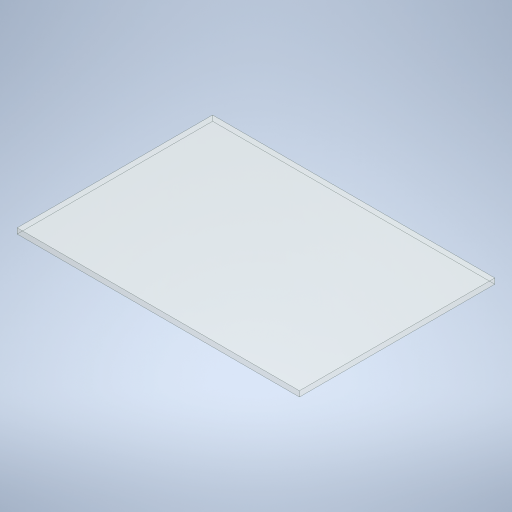
# Autodesk Inventor part: panel_13x9
Saved by Autodesk Inventor 2024 (Build 280153000, 153)
## iProperties
Created: 2024-09-19
Part Number: panel_13x9
Material: Glass
Document SubType Name: Modeling
Designer: Owner
Density: 2.18 g/cm^3
Appearance: Clear
Author: Owner
Autodesk Inventor part; units mm, degrees
ref_plane "YZ Plane" through (0, 0, 0) normal (1, 0, 0) x (0, 1, 0)
ref_plane "XZ Plane" through (0, 0, 0) normal (0, 1, 0) x (-1, 0, 0)
ref_plane "XY Plane" through (0, 0, 0) normal (0, 0, 1) x (1, 0, 0)
sketch "Sketch1" plane through (0, 0, 0) normal (0, 1, 0) x (-1, 0, 0)
  line L0 (165.1, 114.3) -> (-165.1, 114.3)
  line L1 (-165.1, 114.3) -> (-165.1, -114.3)
  line L2 (-165.1, -114.3) -> (165.1, -114.3)
  line L3 (165.1, -114.3) -> (165.1, 114.3)
  line L4 (165.1, 114.3) -> (-165.1, -114.3) construction
  line L5 (-165.1, 114.3) -> (165.1, -114.3) construction
  point P0 (0, 0)
  dimension "d0" = 330.2
  dimension "d1" = 228.6
  constraints: 12 end point, 2 midpoint, 2 parallel, 1 horizontal, 1 perpendicular
  measures "d0" distance of L2.end L1.end
  measures "d1" distance of L1.end L0.end
extrude "Extrusion1" add sketch "Sketch1" along normal blind 6.35
body "Solid1"
